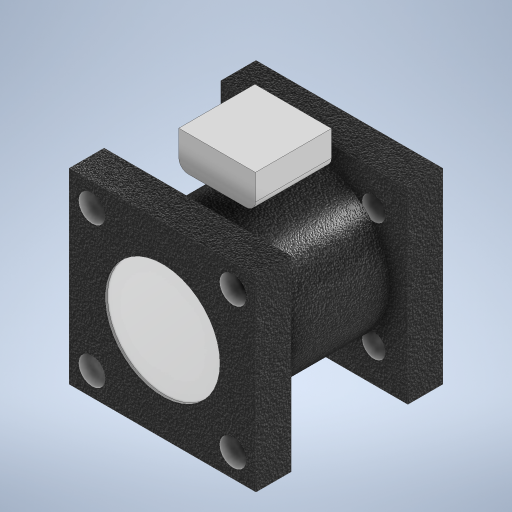
# Autodesk Inventor part: sensor_AMTI
Saved by Autodesk Inventor 2024 (Build 280153000, 153)
## iProperties
Created: 2024-08-07
Part Number: sensor_AMTI
Material: Generic
Document SubType Name: Modeling
Designer: maint
Density: 1 g/cm^3
Appearance: Default
Author: maint
Autodesk Inventor part; units mm, degrees
ref_plane "YZ Plane" through (0, 0, 0) normal (1, 0, 0) x (0, 1, 0)
ref_plane "XZ Plane" through (0, 0, 0) normal (0, 1, 0) x (-1, 0, 0)
ref_plane "XY Plane" through (0, 0, 0) normal (0, 0, 1) x (1, 0, 0)
sketch "Sketch1" plane through (0, 0, 0) normal (0, 0, 1) x (1, 0, 0)
  line L0 (40, -40) -> (-40, -40)
  line L1 (-40, -40) -> (-40, 40)
  line L2 (-40, 40) -> (40, 40)
  line L3 (40, 40) -> (40, -40)
  line L4 (40, -40) -> (-40, 40) construction
  line L5 (-40, -40) -> (40, 40) construction
  point P0 (0, 0)
  dimension "d2" = 80
  constraints: 12 end point, 2 midpoint, 2 parallel, 2 perpendicular, 1 horizontal
  measures "d2" distance of L1.end L2.end
extrude "Extrusion1" add sketch "Sketch1" along normal blind 15
sketch "Sketch2" plane through (0, 0, 15) normal (0, 0, 1) x (1, 0, 0)
  circle A0 centre (0, 0) radius 31.75
  dimension "d21" = 63.5
  constraints: 1 centre point, 1 coincident
  measures "d21" diameter of A0
extrude "Extrusion2" add sketch "Sketch2" along normal blind 50
sketch "Sketch3" plane through (0, 0, 65) normal (0, 0, 1) x (1, 0, 0)
  line L0 (-40, 40) -> (-40, -40) projected
  line L1 (40, -40) -> (-40, -40)
  line L2 (-40, -40) -> (-40, 40)
  line L3 (-40, 40) -> (40, 40)
  line L4 (40, 40) -> (40, -40)
  line L5 (40, -40) -> (-40, 40) construction
  line L6 (-40, -40) -> (40, 40) construction
  point P0 (0, 0)
  constraints: 12 end point, 2 midpoint, 2 parallel, 1 horizontal, 1 perpendicular
extrude "Extrusion3" add sketch "Sketch3" along normal blind 15
sketch "Sketch4" plane through (-40, 40, 0) normal (0, 1, 0) x (1, 0, 0)
  line L0 (56.3965, -56.6426) -> (23.6035, -56.6426)
  line L1 (23.6035, -56.6426) -> (23.6035, -24.0788)
  line L2 (23.6035, -24.0788) -> (56.3965, -24.0788)
  line L3 (56.3965, -24.0788) -> (56.3965, -56.6426)
  line L4 (56.3965, -56.6426) -> (23.6035, -24.0788) construction
  line L5 (23.6035, -56.6426) -> (56.3965, -24.0788) construction
  point P0 (40, 0)
  point P1 (40, -40.3607)
  constraints: 12 end point, 2 midpoint, 2 parallel, 1 horizontal, 1 perpendicular
extrude "Extrusion4" add sketch "Sketch4" along normal blind 15
fillet "Fillet1" radius 4 1 edges at (-16.3965, 40, 40.3607)
fillet "Fillet2" radius 4 1 edges at (16.3965, 40, 40.3607)
sketch "Sketch5" plane through (-40, -40, 65) normal (0, -1, 0) x (1, 0, 0)
  line L0 (52.5319, -29.4542) -> (3.369, -28.3729) construction
  line L1 (3.369, -28.3729) -> (3.6465, -15.7537) construction
  line L2 (3.6465, -15.7537) -> (52.8094, -16.835) construction
  line L3 (52.8094, -16.835) -> (52.5319, -29.4542) construction
  line L4 (52.6907, -23.3562) -> (50.4957, -29.4094)
  line L5 (50.4957, -29.4094) -> (48.8253, -29.3727)
  line L6 (48.8253, -29.3727) -> (46.8986, -23.2288)
  line L7 (46.8986, -23.2288) -> (48.4751, -23.2635)
  line L8 (48.4751, -23.2635) -> (48.8283, -24.5173)
  line L9 (48.8283, -24.5173) -> (50.7458, -24.5595)
  line L10 (50.7458, -24.5595) -> (51.1587, -23.3225)
  line L11 (51.1587, -23.3225) -> (52.6907, -23.3562)
  line L12 (49.14, -25.6317) -> (49.7184, -27.6618)
  line L13 (49.7184, -27.6618) -> (50.3903, -25.6592)
  line L14 (50.3903, -25.6592) -> (49.14, -25.6317)
  line L15 (40.0637, -23.0785) -> (41.5859, -23.112)
  line L16 (41.5859, -23.112) -> (41.497, -27.1546)
  line L17 (41.497, -27.1546) -> (42.6614, -24.5695)
  line L18 (42.6614, -24.5695) -> (43.7091, -24.5926)
  line L19 (43.7091, -24.5926) -> (44.7587, -27.2264)
  line L20 (44.7587, -27.2264) -> (44.8477, -23.1837)
  line L21 (44.8477, -23.1837) -> (46.2907, -23.2155)
  line L22 (46.2907, -23.2155) -> (46.1566, -29.314)
  line L23 (46.1566, -29.314) -> (44.3923, -29.2752)
  line L24 (44.3923, -29.2752) -> (43.1043, -26.2357)
  line L25 (43.1043, -26.2357) -> (41.6939, -29.2158)
  line L26 (41.6939, -29.2158) -> (39.9296, -29.177)
  line L27 (39.9296, -29.177) -> (40.0637, -23.0785)
  line L28 (37.6273, -23.0249) -> (37.5187, -27.9621)
  line L29 (37.5187, -27.9621) -> (39.3225, -28.0017)
  line L30 (39.3225, -28.0017) -> (39.297, -29.1631)
  line L31 (39.297, -29.1631) -> (34.1572, -29.0501)
  line L32 (34.1572, -29.0501) -> (34.1828, -27.8887)
  line L33 (34.1828, -27.8887) -> (35.9866, -27.9284)
  line L34 (35.9866, -27.9284) -> (36.0952, -22.9912)
  line L35 (36.0952, -22.9912) -> (37.6273, -23.0249)
  line L36 (30.6293, -22.871) -> (33.9108, -22.9432)
  line L37 (33.9108, -22.9432) -> (33.8875, -24.0057)
  line L38 (33.8875, -24.0057) -> (33.0127, -23.9865)
  line L39 (33.0127, -23.9865) -> (32.9253, -27.9599)
  line L40 (32.9253, -27.9599) -> (33.8001, -27.9792)
  line L41 (33.8001, -27.9792) -> (33.7767, -29.0417)
  line L42 (33.7767, -29.0417) -> (30.4952, -28.9695)
  line L43 (30.4952, -28.9695) -> (30.5185, -27.907)
  line L44 (30.5185, -27.907) -> (31.3933, -27.9262)
  line L45 (31.3933, -27.9262) -> (31.4807, -23.9528)
  line L46 (31.4807, -23.9528) -> (30.6059, -23.9336)
  line L47 (30.6059, -23.9336) -> (30.6293, -22.871)
  point P0 (40, -65)
  constraints: 2 other
extrude "Extrusion5" add sketch "Sketch5" against normal blind 2
sketch "Sketch6" plane through (0, 0, 80) normal (0, 0, 1) x (1, 0, 0)
  circle A0 centre (0, 0) radius 24.5699
  constraints: 1 centre point, 1 coincident
extrude "Extrusion6" cut sketch "Sketch6" against normal blind 1
sketch "Sketch7" plane through (0, 0, 80) normal (0, 0, 1) x (1, 0, 0)
  circle A0 centre (30.1625, -30.1625) radius 5.7961
  circle A1 centre (-30.1625, -30.1625) radius 5.7961
  circle A2 centre (-30.1625, 30.1625) radius 5.7961
  circle A3 centre (30.1625, 30.1625) radius 5.7961
  line L0 (30.1625, 30.1625) -> (-30.1625, 30.1625)
  line L1 (-30.1625, 30.1625) -> (-30.1625, -30.1625)
  line L2 (-30.1625, -30.1625) -> (30.1625, -30.1625)
  line L3 (30.1625, -30.1625) -> (30.1625, 30.1625)
  line L4 (30.1625, 30.1625) -> (-30.1625, -30.1625) construction
  line L5 (-30.1625, 30.1625) -> (30.1625, -30.1625) construction
  point P0 (0, 0)
  dimension "d22" = 60.325
  constraints: 12 end point, 4 centre point, 4 coincident, 2 midpoint, 2 parallel, 2 perpendicular, 1 horizontal
  measures "d22" distance of L0.end L1.end
extrude "Extrusion7" cut sketch "Sketch7" against normal up to surface (15 mm away) contours A0 L2 L3 | L3 L2 A0 | L3 L0 A3 | A3 L0 L3 | L2 L1 A1 | A1 L1 L2 | L0 L1 A2 | A2 L1 L0
sketch "Sketch8" plane through (0, 0, 0) normal (0, 0, -1) x (-1, 0, 0)
  line L0 (25.4, -25.4) -> (-25.4, -25.4)
  line L1 (-25.4, -25.4) -> (-25.4, 25.4)
  line L2 (-25.4, 25.4) -> (25.4, 25.4)
  line L3 (25.4, 25.4) -> (25.4, -25.4)
  line L4 (25.4, -25.4) -> (-25.4, 25.4) construction
  line L5 (-25.4, -25.4) -> (25.4, 25.4) construction
  circle A0 centre (25.4, 25.4) radius 5.08
  circle A1 centre (25.4, -25.4) radius 5.08
  circle A2 centre (-25.4, -25.4) radius 5.08
  circle A3 centre (-25.4, 25.4) radius 5.08
  point P0 (0, 0)
  dimension "d19" = 50.8
  dimension "d20" = 10.16
  constraints: 12 end point, 4 centre point, 4 coincident, 3 equal radius, 2 midpoint, 2 parallel, 2 perpendicular, 1 horizontal
  measures "d19" distance of L1.end L2.end
  measures "d20" diameter of A1
extrude "Extrusion8" cut sketch "Sketch8" against normal up to surface (15 mm away) contours A2 L1 L0 | L0 L1 A2 | A1 L3 L0 | L0 L3 A1 | A3 L2 L1 | L1 L2 A3 | A0 L2 L3 | L3 L2 A0
body "Solid1"
